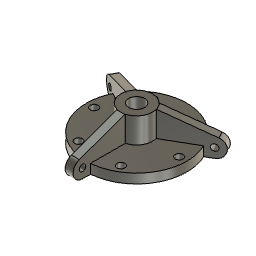
A3_AI22BTECH11005_1 (Autodesk Fusion 360 design; units mm, degrees)
Autodesk Fusion 360 part; units mm, degrees
note: some values were not read from the file. Set by a fixed rule: which sketch regions a step uses.
sketch "Sketch1" plane through (0, 0, 0) normal (0, 0, 1) x (1, 0, 0)
  circle A0 centre (0, 0) radius 101.5
  circle A1 centre (0, 0) radius 16
  circle A2 centre (0, 0) radius 32
  dimension "d1" = 203
  dimension "d2" = 32
  dimension "d3" = 64
  constraint coincident A0.centre A1.centre
  constraint concentric A1 A2
  measures "d1" diameter of A0
  measures "d2" diameter of A1
  measures "d3" diameter of A2
extrude "Extrude1" add sketch "Sketch1" along normal blind 51 contours A2
extrude "Extrude2" add sketch "Sketch1" against normal blind 19 contours A0 | A1 | A2
sketch "Sketch2" plane through (0, 0, 0) normal (0, 0, 1) x (1, 0, 0)
  circle A0 centre (0, 0) radius 86
  circle A1 centre (0, 0) radius 32
  circle A2 centre (0, 0) radius 101.5
  circle A3 centre (0, 0) radius 32
  circle A4 centre (-85.9999, 0.1299) radius 8
  dimension "d8" = 172
  dimension "d9" = 64
  dimension "d10" = 64
  dimension "d11" = 203
  dimension "d12" = 64
  dimension "d13" = 16
  constraint coincident A0.centre A1.centre
  constraint coincident A0 A4.centre
  measures "d8" diameter of A0
  measures "d9" diameter of A1
  measures "d10" diameter of A1
  measures "d11" diameter of A2
  measures "d12" diameter of A3
  measures "d13" diameter of A4
extrude "Extrude3" cut sketch "Sketch2" against normal blind 30 contours A0 A4 | A0 A4 picked at (-83.3057, 0.1299) picked at (-88.639, 0.1339)
pattern_circular "C-Pattern1" count 6 over 360 about axis through (0, 0, 1.75) along (0, 0, 1) of "Extrude3"
ref_plane "WorkPlane2" through (-117.5, 0, 4.8107) normal (-1, 0, 0) x (0, 1, 0)
ref_plane "WorkPlane3" through (0, 0, 4.8107) normal (-1, 0, 0) x (0, 1, 0)
sketch "Sketch7" plane through (0, 0, 0) normal (0, 0, 1) x (1, 0, 0)
  line L0 (0, 0) -> (0, -117.5)
  circle A0 centre (0, -117.5) radius 6.5
  dimension "d26" = 117.5
  dimension "d27" = 13
  constraint coincident L0.start origin
  constraint vertical L0
  constraint coincident L0.end A0.centre
  measures "d26" distance of L0.start L0.end
  measures "d27" diameter of A0
extrude "Extrude7" cut sketch "Sketch7" along normal mid plane 16
sketch "Sketch10" plane through (0, 0, 0) normal (1, 0, 0) x (0, 1, 0)
  line L0 (0, 0) -> (-117.5, 0)
  circle A0 centre (-117.5, 0) radius 6.5
  circle A1 centre (-117.5, 0) radius 19
  circle A2 centre (-117.5, 0) radius 6.5
  dimension "d28" = 117.5
  dimension "d29" = 13
  dimension "d30" = 38
  constraint coincident L0.start origin
  constraint horizontal L0
  constraint coincident L0.end A0.centre
  constraint concentric A0 A1
  constraint concentric A1 A2
  measures "d28" distance of L0.start L0.end
  measures "d29" diameter of A0
  measures "d30" diameter of A1
sketch "Sketch12" plane through (0, 0, 0) normal (1, 0, 0) x (0, 1, 0)
  line L0 (0, 0) -> (0, 51)
  line L1 (-123.9402, 17.8752) -> (-124.2542, 17.7621)
  circle A0 centre (-117.5, 0) radius 19
  line L2 (-32, 0) -> (-117.5, 0)
  line L3 (-117.5, 0) -> (-117.5, -10)
  line L4 (-117.5, -10) -> (-133.6555, -10)
  line L5 (-32, 51) -> (-123.9402, 17.8752)
  arc A1 (-98.5, 0) -> (-123.9402, 17.8752) centre (-117.5, 0) ccw
  arc A2 (-123.9402, 17.8752) -> (-133.6555, -10) centre (-117.5, 0) ccw
  line L6 (-32, 51) -> (-25, 51)
  line L7 (-25, 51) -> (-25, 0)
  line L8 (-25, 0) -> (-50, 0)
  line L9 (-25, 0) -> (-25, -19)
  line L10 (-25, -19) -> (-117.5, -19)
  dimension "d31" = 51
  dimension "d33" = 51
  dimension "d40" = 19
  constraint coincident L0.start origin
  constraint vertical L0
  constraint tangent L1 A0
  constraint coincident A0.centre L2.end
  constraint perpendicular L2 L3
  constraint perpendicular L3 L4
  constraint coincident A0 L1.start
  constraint tangent A0 L5
  constraint coincident A0 L4.end
  constraint concentric A1 A2
  constraint coincident L2 A1.start
  constraint horizontal L6
  constraint perpendicular L6 L7
  constraint coincident L2 L8.end
  constraint perpendicular L7 L8
  constraint perpendicular L8 L9
  constraint coincident A0 L10.end
  constraint tangent A0 L10
  constraint perpendicular L9 L10
  measures "d31" distance of L0.start L0.end
  measures "d33" distance of L5.start L2.start
  measures "d40" distance of L7.end L9.end
extrude "Extrude9" add sketch "Sketch12" along normal mid plane 16
extrude "Extrude8" cut sketch "Sketch10" along normal mid plane 16 contours A0 A2
pattern_circular "C-Pattern2" count 3 over 360 about axis through (0, 0, 0) along (0, 0, 1) of "Extrude9", "Extrude8"
named bodies: "base"
